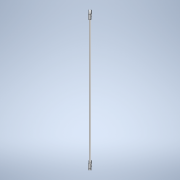
# Autodesk Inventor part: 04_10 Cable
Saved by Autodesk Inventor 2021 (Build 250183000, 183)
## iProperties
Created: 2021-06-25
Part Number: 04_10 Cable
Material: Genérico
Document SubType Name: Modeling
Designer: Almanzor
Density: 1 g/cm^3
Appearance: Valor por defecto
Author: Almanzor
Autodesk Inventor part; units mm, degrees
ref_plane "YZ Plane" through (0, 0, 0) normal (1, 0, 0) x (0, 1, 0)
ref_plane "XZ Plane" through (0, 0, 0) normal (0, 1, 0) x (-1, 0, 0)
ref_plane "XY Plane" through (0, 0, 0) normal (0, 0, 1) x (1, 0, 0)
sketch "Boceto1" plane through (0, 0, 0) normal (0, 1, 0) x (-1, 0, 0)
  circle A0 centre (0, 0) radius 8.5
  dimension "d0" = 17
  constraints: 1 centre point, 1 coincident
  measures "d0" diameter of A0
extrude "Extrusión1" add sketch "Boceto1" along normal blind 1500
sketch "Boceto2" plane through (0, 1500, 0) normal (0, 1, 0) x (1, 0, 0)
  line L0 (24.0008, -12.205) -> (-8.9626, 25.3904)
  line L1 (-8.9626, 25.3904) -> (-24.0008, 12.205)
  line L2 (-24.0008, 12.205) -> (8.9626, -25.3904)
  line L3 (8.9626, -25.3904) -> (24.0008, -12.205)
  line L4 (24.0008, -12.205) -> (-24.0008, 12.205) construction
  line L5 (-8.9626, 25.3904) -> (8.9626, -25.3904) construction
  point P0 (0, 0)
  dimension "d3" = 20
  dimension "d4" = 50
  constraints: 12 end point, 2 midpoint, 2 parallel, 1 perpendicular
  measures "d3" distance of L0.end L1.end
  measures "d4" distance of L0.start L0.end
extrude "Extrusión2" add sketch "Boceto2" along normal blind 80
sketch "Boceto3" plane through (-8.9626, 1500, -25.3904) normal (0.7519079, 0, -0.6592681) x (-0.6592681, 0, -0.7519079)
  circle A0 centre (-25, 55) radius 8.5
  line L0 (-50, 80) -> (0, 80) projected
  line L1 (0, 0) -> (0, 80) projected
  point P0 (-25, -1500)
  dimension "d7" = 17
  dimension "d8" = 25
  dimension "d9" = 25
  constraints: 1 centre point
  measures "d7" diameter of A0
  measures "d8" distance from line of L0 A0.centre
  measures "d9" distance from line of L1 A0.centre
extrude "Extrusión3" cut sketch "Boceto3" against normal blind 80
fillet "Empalme1" radius 25 2 edges at (-16.4817, 1580, -18.7977) (16.4817, 1580, 18.7977)
sketch "Boceto4" plane through (0, 0, 0) normal (0, -1, 0) x (1, 0, 0)
  line L0 (-8.9626, -25.3904) -> (-24.0008, -12.205) projected
  line L1 (24.0008, 12.205) -> (-8.9626, -25.3904) projected
  line L2 (8.9626, 25.3904) -> (24.0008, 12.205) projected
  line L3 (-24.0008, -12.205) -> (8.9626, 25.3904) projected
  circle A0 centre (0, 0) radius 8.5 projected
  line L4 (24.0008, 12.205) -> (-8.9626, -25.3904) projected
  line L5 (24.0008, 12.205) -> (-8.9626, -25.3904)
  line L6 (-8.9626, -25.3904) -> (-24.0008, -12.205) projected
  line L7 (-8.9626, -25.3904) -> (-24.0008, -12.205)
  line L8 (-24.0008, -12.205) -> (8.9626, 25.3904) projected
  line L9 (-24.0008, -12.205) -> (8.9626, 25.3904)
  line L10 (8.9626, 25.3904) -> (24.0008, 12.205) projected
  line L11 (8.9626, 25.3904) -> (24.0008, 12.205)
  constraints: 8 end point, 4 collinear
extrude "Extrusión4" add sketch "Boceto4" along normal blind 80 contours L0 L3 L2 L1 | A0
sketch "Boceto5" plane through (24.0008, -80, 12.205) normal (0.7519079, 0, -0.6592681) x (-0.6592681, 0, -0.7519079)
  circle A0 centre (25, 25) radius 8.5
  line L0 (0, 80) -> (0, 0) projected
  line L1 (50, 0) -> (0, 0) projected
  point P0 (25, 80)
  dimension "d15" = 17
  dimension "d16" = 25
  dimension "d17" = 25
  constraints: 1 centre point
  measures "d15" diameter of A0
  measures "d16" distance from line of L0 A0.centre
  measures "d17" distance from line of L1 A0.centre
extrude "Extrusión5" cut sketch "Boceto5" against normal blind 80
fillet "Empalme2" radius 25 2 edges at (-16.4817, -80, -18.7977) (16.4817, -80, 18.7977)
